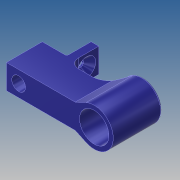
# Autodesk Inventor part: KB33-046-003-001 - Крепление
Saved by Autodesk Inventor 2020 (Build 240168000, 168)
## iProperties
Created: 2021-06-09
Part Number: KB33-046-003-001 - Крепление
Material: ABS Plastic
Document SubType Name: Modeling
Designer: Петров Иван
Density: 1.06 g/cm^3
Appearance: Smooth - Navy
Mass: 198.18 g
Surface Area: 401.565 cm^2
Volume: 186.962 cm^3
Author: Петров Иван
Autodesk Inventor part; units mm, degrees
ref_plane "XZ Plane" through (0, 0, 0) normal (0, 1, 0) x (-1, 0, 0)
ref_plane "XY Plane" through (0, 0, 0) normal (0, 0, 1) x (1, 0, 0)
sketch "Sketch1" plane through (0, 0, 0) normal (0, 0, 1) x (1, 0, 0)
  circle A0 centre (0, 0) radius 19.25
  circle A1 centre (0, 0) radius 25
  dimension "d0" = 38.5
  dimension "d1" = 50
  constraints: 2 centre point, 2 coincident
  measures "d0" diameter of A0
  measures "d1" diameter of A1
extrude "Extrusion1" add sketch "Sketch1" along normal blind 60
sketch "Sketch2" plane through (0, 0, 0) normal (0, 0, -1) x (-1, 0, 0)
  circle A0 centre (0, 0) radius 25
  arc A1 (-9.9286, -5.8029) -> (-9.9286, 5.8029) centre (0, 0) ccw
  arc A2 (-9.9286, 5.8029) -> (-9.9286, -5.8029) centre (-7, 0) ccw
  circle A3 centre (0, -15) radius 1.25
  circle A4 centre (12.9904, -7.5) radius 1.25
  circle A5 centre (12.9904, 7.5) radius 1.25
  circle A6 centre (0, 15) radius 1.25
  circle A7 centre (-12.9904, 7.5) radius 1.25
  circle A8 centre (-12.9904, -7.5) radius 1.25
  circle A9 centre (-7, 0) radius 6
  arc A10 (-10.375, -4.9608) -> (-10.375, 4.9608) centre (-7, 0) ccw
  spline S0 degree 3 poles (-10.375, 4.9608) (-10.4487, 4.9106) (-10.5225, 4.858) (-10.5964, 4.8027) knots 0 0 0 0 1 1 1 1
  arc A11 (-10.5964, 4.8027) -> (-10.5964, -4.8027) centre (-7, 0) ccw
  spline S1 degree 3 poles (-10.5964, -4.8027) (-10.5225, -4.858) (-10.4487, -4.9106) (-10.375, -4.9608) knots 0 0 0 0 1 1 1 1
  dimension "d4" = 50
  constraints: 12 centre point, 8 point on circle, 37 other
  measures "d4" diameter of A0
extrude "Extrusion2" add sketch "Sketch2" along normal blind 4 contours A0 | A2 A1
sketch "Sketch3" plane through (0, 0, -4) normal (0, 0, -1) x (-1, 0, 0)
  arc A0 (-10.375, -4.9608) -> (-10.375, 4.9608) centre (-7, 0) ccw projected
  circle A1 centre (-7, 0) radius 6.5
  point P0 (0, 0)
  dimension "d7" = 13
  constraints: 1 centre point, 1 coincident
  measures "d7" diameter of A1
extrude "Extrusion3" cut sketch "Sketch3" against normal blind 4
ref_plane "Work Plane1" through (-25, 0, 0) normal (1, 0, 0) x (0, 1, 0)
sketch "Sketch5" plane through (0, 0, 60) normal (0, 0, 1) x (1, 0, 0)
  circle A0 centre (0, 0) radius 25 projected
  line L0 (-19.2094, -16) -> (-25, -16)
  line L1 (-25, -16) -> (-25, 16)
  line L2 (-25, 16) -> (-19.2094, 16)
  circle A1 centre (0, 0) radius 19.25 projected
  line L3 (-19.2094, 16) -> (-19.2094, 1.25)
  line L4 (-19.2094, -1.25) -> (-19.2094, -16)
  dimension "d84" = 32
  constraints: 10 end point, 4 point on circle, 3 parallel, 1 horizontal, 1 perpendicular, 1 tangent
  measures "d84" distance of L0.end L1.end
extrude "Extrusion4" add sketch "Sketch5" against normal blind 40 contours L3 A1 L4 A0 | A0 L1 L2 | L0 L1 A0 picked at (-20.2622, -9.4719)
fillet "Сопряжение13" radius 386.75 2 edges at (-19.2094, -16, 40) (-19.2094, 16, 40)
fillet "Сопряжение15" radius 2 1 edges at (25, 0, -4)
sketch "Эскиз15" plane through (-25, -16, 60) normal (-1, 0, 0) x (0, 0, 1)
  line L0 (0, 32) -> (0, 0) projected
  line L1 (0, 32) -> (-40, 32) projected
  line L2 (-40, 16) -> (-40, 32) projected
  line L3 (-40, 0) -> (-40, 16) projected
  line L4 (0, 0) -> (-40, 0) projected
  point P0 (-60, 16)
extrude "Выдавливание11" add sketch "Эскиз15" along normal blind 90
fillet "Сопряжение16" radius 21.25 1 edges at (-25, 0, 20)
sketch "Эскиз16" plane through (0, 0, 20) normal (0, 0, -1) x (-1, 0, 0)
  line L0 (25, 16) -> (115, 16) projected
  line L1 (25, -16) -> (115, -16) projected
  line L2 (115, 16) -> (83, 16)
  line L3 (83, 16) -> (83, -16)
  line L4 (83, -16) -> (115, -16)
  line L5 (115, -16) -> (115, 16)
  point P0 (0, 0)
  point P1 (83, 16)
  dimension "d57" = 32
  constraints: 8 end point, 2 parallel, 1 horizontal, 1 perpendicular, 1 point on line
  measures "d57" distance of L4.end L3.end
extrude "Выдавливание12" add sketch "Эскиз16" along normal blind 7
sketch "Эскиз17" plane through (0, 0, 20) normal (0, 0, -1) x (-1, 0, 0)
  line L0 (43.3943, 16) -> (83, 16) projected
  line L1 (43.3943, -16) -> (83, -16) projected
  line L2 (83, 16) -> (73, 16)
  line L3 (73, 16) -> (73, -16)
  line L4 (73, -16) -> (83, -16)
  line L5 (83, -16) -> (83, 16)
  point P0 (0, 0)
  dimension "d62" = 10
  constraints: 8 end point, 2 parallel, 1 horizontal, 1 perpendicular, 1 point on line
  measures "d62" distance of L4.end L3.end
extrude "Выдавливание13" add sketch "Эскиз17" along normal blind 39
fillet "Сопряжение19" radius 2.5 1 edges at (-83, 0, 13)
sketch "Эскиз18" plane through (-83, -16, -19) normal (-1, 0, 0) x (0, 0, 1)
  line L0 (0, 32) -> (0, 0) projected
  line L1 (0, 16) -> (16, 16) construction
  circle A0 centre (16, 16) radius 4
  dimension "d88" = 16
  dimension "d89" = 8
  constraints: 2 end point, 1 centre point, 1 coincident, 1 horizontal, 1 midpoint
  measures "d88" distance of L1.start L1.end
  measures "d89" diameter of A0
sketch "Эскиз19" plane through (0, 0, 13) normal (0, 0, -1) x (-1, 0, 0)
  circle A0 centre (99, 0) radius 4
  line L0 (115, -16) -> (115, 16) projected
  point P0 (0, 0)
  point P1 (115, -13.5)
  point P2 (115, 13.5)
  dimension "d85" = 8
  dimension "d86" = 16
  constraints: 1 centre point
  measures "d85" diameter of A0
  measures "d86" distance from line of A0.centre L0
extrude "Выдавливание14" cut sketch "Эскиз19" against normal blind 90
extrude "Выдавливание15" cut sketch "Эскиз18" against normal blind 19.75
chamfer "Фаска3" distance 8 angle 45 1 edges at (-73, 0, -7)
fillet "Сопряжение20" radius 12.25 1 edges at (-73, 0, 20)
ref_plane "РабПлоскость4" through (0, 25, 0) normal (0, 1, 0) x (-1, 0, 0)
sketch "Эскиз22" plane through (0, 25, 0) normal (0, 1, 0) x (-1, 0, 0)
  line L0 (98.8193, 69.0383) -> (98.8193, 37.0439)
  line L1 (98.8193, 37.0439) -> (0, 37.0439)
  line L2 (0, 37.0439) -> (0, 60)
  line L3 (-19.25, 60) -> (19.25, 60) projected
  point P0 (0, 0)
  constraints: 6 end point, 1 midpoint, 1 perpendicular, 1 vertical
sketch "Эскиз25" plane through (0, 0, 60) normal (0, 0, 1) x (1, 0, 0)
  circle A0 centre (-99, 0) radius 4 projected
  circle A1 centre (-99, 0) radius 9
  point P0 (0, 0)
  dimension "d98" = 18
  constraints: 1 centre point, 1 coincident
  measures "d98" diameter of A1
extrude "Выдавливание17" cut sketch "Эскиз25" against normal blind 32
chamfer "Фаска5" distance 5 angle 45 1 edges at (-95, 0, 28)
body "Solid1"
